Autodesk Fusion 360 part; units mm, degrees
(part 4 of 7)
  line L871 (67.0056, -68.9388) -> (67.1048, -68.852)
  line L872 (67.1048, -68.852) -> (67.2027, -68.7638)
  line L873 (67.2027, -68.7638) -> (67.2994, -68.6742)
  line L874 (67.2994, -68.6742) -> (67.2738, -68.5996)
  line L875 (67.2738, -68.5996) -> (67.2468, -68.526)
  line L876 (67.2468, -68.526) -> (67.2184, -68.4537)
  line L877 (67.2184, -68.4537) -> (67.1886, -68.3826)
  line L878 (67.1886, -68.3826) -> (67.1574, -68.3128)
  line L879 (67.1574, -68.3128) -> (67.1246, -68.2444)
  line L880 (67.1246, -68.2444) -> (67.0902, -68.1774)
  line L881 (67.0902, -68.1774) -> (67.0542, -68.1121)
  line L882 (67.0542, -68.1121) -> (67.0162, -68.0485)
  line L883 (67.0162, -68.0485) -> (66.9762, -67.987)
  line L884 (66.9762, -67.987) -> (66.9336, -67.9279)
  line L885 (66.9336, -67.9279) -> (66.8873, -67.8725)
  line L886 (66.8873, -67.8725) -> (66.5717, -67.5557)
  line L887 (66.5717, -67.5557) -> (66.7231, -67.4007)
  line L888 (66.7231, -67.4007) -> (66.8702, -67.2417)
  line L889 (66.8702, -67.2417) -> (67.013, -67.0787)
  line L890 (67.013, -67.0787) -> (67.1514, -66.9119)
  line L891 (67.1514, -66.9119) -> (67.4994, -67.1928)
  line L892 (67.4994, -67.1928) -> (67.5593, -67.233)
  line L893 (67.5593, -67.233) -> (67.6225, -67.2692)
  line L894 (67.6225, -67.2692) -> (67.6879, -67.3025)
  line L895 (67.6879, -67.3025) -> (67.7551, -67.3336)
  line L896 (67.7551, -67.3336) -> (67.8238, -67.3627)
  line L897 (67.8238, -67.3627) -> (67.894, -67.3899)
  line L898 (67.894, -67.3899) -> (67.9655, -67.4153)
  line L899 (67.9655, -67.4153) -> (68.0382, -67.4391)
  line L900 (68.0382, -67.4391) -> (68.112, -67.4613)
  line L901 (68.112, -67.4613) -> (68.1869, -67.4819)
  line L902 (68.1869, -67.4819) -> (68.2629, -67.5011)
  line L903 (68.2629, -67.5011) -> (68.3398, -67.5188)
  line L904 (68.3398, -67.5188) -> (68.4187, -67.4133)
  line L905 (68.4187, -67.4133) -> (68.4962, -67.3066)
  line L906 (68.4962, -67.3066) -> (68.5722, -67.1989)
  line L907 (68.5722, -67.1989) -> (68.5316, -67.1312)
  line L908 (68.5316, -67.1312) -> (68.4899, -67.0649)
  line L909 (68.4899, -67.0649) -> (68.4471, -67.0001)
  line L910 (68.4471, -67.0001) -> (68.4032, -66.9367)
  line L911 (68.4032, -66.9367) -> (68.3581, -66.8749)
  line L912 (68.3581, -66.8749) -> (68.3118, -66.8148)
  line L913 (68.3118, -66.8148) -> (68.2643, -66.7565)
  line L914 (68.2643, -66.7565) -> (68.2154, -66.7001)
  line L915 (68.2154, -66.7001) -> (68.1651, -66.6458)
  line L916 (68.1651, -66.6458) -> (68.1131, -66.5939)
  line L917 (68.1131, -66.5939) -> (68.0592, -66.545)
  line L918 (68.0592, -66.545) -> (68.0024, -66.5004)
  line L919 (68.0024, -66.5004) -> (67.6277, -66.2562)
  line L920 (67.6277, -66.2562) -> (67.7436, -66.0731)
  line L921 (67.7436, -66.0731) -> (67.8545, -65.8869)
  line L922 (67.8545, -65.8869) -> (67.9603, -65.6978)
  line L923 (67.9603, -65.6978) -> (68.0609, -65.5059)
  line L924 (68.0609, -65.5059) -> (68.4598, -65.7083)
  line L925 (68.4598, -65.7083) -> (68.5267, -65.7352)
  line L926 (68.5267, -65.7352) -> (68.5961, -65.7574)
  line L927 (68.5961, -65.7574) -> (68.667, -65.7765)
  line L928 (68.667, -65.7765) -> (68.7391, -65.7929)
  line L929 (68.7391, -65.7929) -> (68.8124, -65.807)
  line L930 (68.8124, -65.807) -> (68.8867, -65.819)
  line L931 (68.8867, -65.819) -> (68.9619, -65.8291)
  line L932 (68.9619, -65.8291) -> (69.038, -65.8372)
  line L933 (69.038, -65.8372) -> (69.1148, -65.8436)
  line L934 (69.1148, -65.8436) -> (69.1924, -65.8482)
  line L935 (69.1924, -65.8482) -> (69.2706, -65.8511)
  line L936 (69.2706, -65.8511) -> (69.3495, -65.8525)
  line L937 (69.3495, -65.8525) -> (69.4049, -65.7328)
  line L938 (69.4049, -65.7328) -> (69.4585, -65.6124)
  line L939 (69.4585, -65.6124) -> (69.5104, -65.4913)
  line L940 (69.5104, -65.4913) -> (69.4566, -65.4335)
  line L941 (69.4566, -65.4335) -> (69.402, -65.3773)
  line L942 (69.402, -65.3773) -> (69.3467, -65.3228)
  line L943 (69.3467, -65.3228) -> (69.2906, -65.2699)
  line L944 (69.2906, -65.2699) -> (69.2336, -65.2189)
  line L945 (69.2336, -65.2189) -> (69.1758, -65.1697)
  line L946 (69.1758, -65.1697) -> (69.1172, -65.1225)
  line L947 (69.1172, -65.1225) -> (69.0577, -65.0775)
  line L948 (69.0577, -65.0775) -> (68.9971, -65.0349)
  line L949 (68.9971, -65.0349) -> (68.9355, -64.9949)
  line L950 (68.9355, -64.9949) -> (68.8726, -64.9583)
  line L951 (68.8726, -64.9583) -> (68.8078, -64.9265)
  line L952 (68.8078, -64.9265) -> (68.3906, -64.7655)
  line L953 (68.3906, -64.7655) -> (68.4658, -64.5623)
  line L954 (68.4658, -64.5623) -> (68.5356, -64.3572)
  line L955 (68.5356, -64.3572) -> (68.5998, -64.1502)
  line L956 (68.5998, -64.1502) -> (68.6583, -63.9416)
  line L957 (68.6583, -63.9416) -> (69.0905, -64.0566)
  line L958 (69.0905, -64.0566) -> (69.1616, -64.069)
  line L959 (69.1616, -64.069) -> (69.234, -64.0763)
  line L960 (69.234, -64.0763) -> (69.3073, -64.0802)
  line L961 (69.3073, -64.0802) -> (69.3814, -64.0813)
  line L962 (69.3814, -64.0813) -> (69.456, -64.0798)
  line L963 (69.456, -64.0798) -> (69.5312, -64.0761)
  line L964 (69.5312, -64.0761) -> (69.6068, -64.0703)
  line L965 (69.6068, -64.0703) -> (69.6829, -64.0625)
  line L966 (69.6829, -64.0625) -> (69.7594, -64.0527)
  line L967 (69.7594, -64.0527) -> (69.8362, -64.0411)
  line L968 (69.8362, -64.0411) -> (69.9133, -64.0277)
  line L969 (69.9133, -64.0277) -> (69.9908, -64.0126)
  line L970 (69.9908, -64.0126) -> (70.02, -63.8841)
  line L971 (70.02, -63.8841) -> (70.0474, -63.7552)
  line L972 (70.0474, -63.7552) -> (70.073, -63.6259)
  line L973 (70.073, -63.6259) -> (70.0084, -63.5805)
  line L974 (70.0084, -63.5805) -> (69.9433, -63.5369)
  line L975 (69.9433, -63.5369) -> (69.8779, -63.4951)
  line L976 (69.8779, -63.4951) -> (69.812, -63.4551)
  line L977 (69.812, -63.4551) -> (69.7457, -63.417)
  line L978 (69.7457, -63.417) -> (69.6789, -63.3809)
  line L979 (69.6789, -63.3809) -> (69.6118, -63.3469)
  line L980 (69.6118, -63.3469) -> (69.5442, -63.3153)
  line L981 (69.5442, -63.3153) -> (69.4761, -63.2861)
  line L982 (69.4761, -63.2861) -> (69.4076, -63.2599)
  line L983 (69.4076, -63.2599) -> (69.3384, -63.2371)
  line L984 (69.3384, -63.2371) -> (69.2684, -63.2195)
  line L985 (69.2684, -63.2195) -> (68.8268, -63.1488)
  line L986 (68.8268, -63.1488) -> (68.8582, -62.9344)
  line L987 (68.8582, -62.9344) -> (68.8837, -62.7192)
  line L988 (68.8837, -62.7192) -> (68.9035, -62.5034)
  line L989 (68.9035, -62.5034) -> (68.9174, -62.2872)
  circle A0 centre (60.9176, -61.8819) radius 2
extrude "Extrude1''" add sketch "Sketch1 (3)" along normal blind 2 separate body makes body 5 in component "CT idler 2"
ref_plane "WorkPlane2" through (0, 0, 41.2) normal (0, 0, 1) x (1, 0, 0) in component "CT idler 2"
sketch "Sketch2 (2)" plane through (0, 0, 41.2) normal (0, 0, 1) x (1, 0, 0) in component "CT idler 2"
  line L0 (63.9717, -62.352) -> (64.2611, -62.3965)
  line L1 (64.2611, -62.3965) -> (64.3324, -62.3976)
  line L2 (64.3324, -62.3976) -> (64.4048, -62.3905)
  line L3 (64.4048, -62.3905) -> (64.478, -62.3776)
  line L4 (64.478, -62.3776) -> (64.5516, -62.3599)
  line L5 (64.5516, -62.3599) -> (64.6256, -62.3378)
  line L6 (64.6256, -62.3378) -> (64.6997, -62.3116)
  line L7 (64.6997, -62.3116) -> (64.774, -62.2814)
  line L8 (64.774, -62.2814) -> (64.8483, -62.2475)
  line L9 (64.8483, -62.2475) -> (64.9224, -62.21)
  line L10 (64.9224, -62.21) -> (64.9964, -62.1689)
  line L11 (64.9964, -62.1689) -> (65.07, -62.1243)
  line L12 (65.07, -62.1243) -> (65.1432, -62.0763)
  line L13 (65.1432, -62.0763) -> (65.1471, -61.9467)
  line L14 (65.1471, -61.9467) -> (65.1471, -61.8171)
  line L15 (65.1471, -61.8171) -> (65.1432, -61.6876)
  line L16 (65.1432, -61.6876) -> (65.07, -61.6396)
  line L17 (65.07, -61.6396) -> (64.9964, -61.595)
  line L18 (64.9964, -61.595) -> (64.9224, -61.5539)
  line L19 (64.9224, -61.5539) -> (64.8483, -61.5163)
  line L20 (64.8483, -61.5163) -> (64.774, -61.4824)
  line L21 (64.774, -61.4824) -> (64.6997, -61.4523)
  line L22 (64.6997, -61.4523) -> (64.6256, -61.4261)
  line L23 (64.6256, -61.4261) -> (64.5516, -61.404)
  line L24 (64.5516, -61.404) -> (64.478, -61.3862)
  line L25 (64.478, -61.3862) -> (64.4048, -61.3734)
  line L26 (64.4048, -61.3734) -> (64.3324, -61.3662)
  line L27 (64.3324, -61.3662) -> (64.2611, -61.3673)
  line L28 (64.2611, -61.3673) -> (63.9717, -61.4119)
  line L29 (63.9717, -61.4119) -> (63.9415, -61.2461)
  line L30 (63.9415, -61.2461) -> (63.9023, -61.0822)
  line L31 (63.9023, -61.0822) -> (63.8543, -60.9206)
  line L32 (63.8543, -60.9206) -> (63.7975, -60.762)
  line L33 (63.7975, -60.762) -> (64.0705, -60.6558)
  line L34 (64.0705, -60.6558) -> (64.1328, -60.6212)
  line L35 (64.1328, -60.6212) -> (64.1919, -60.5788)
  line L36 (64.1919, -60.5788) -> (64.2488, -60.5311)
  line L37 (64.2488, -60.5311) -> (64.3037, -60.4789)
  line L38 (64.3037, -60.4789) -> (64.3567, -60.4227)
  line L39 (64.3567, -60.4227) -> (64.4079, -60.3629)
  line L40 (64.4079, -60.3629) -> (64.4571, -60.2997)
  line L41 (64.4571, -60.2997) -> (64.5045, -60.2332)
  line L42 (64.5045, -60.2332) -> (64.5499, -60.1636)
  line L43 (64.5499, -60.1636) -> (64.5934, -60.0911)
  line L44 (64.5934, -60.0911) -> (64.6348, -60.0156)
  line L45 (64.6348, -60.0156) -> (64.6742, -59.9375)
  line L46 (64.6742, -59.9375) -> (64.6129, -59.8233)
  line L47 (64.6129, -59.8233) -> (64.5481, -59.7111)
  line L48 (64.5481, -59.7111) -> (64.4799, -59.6008)
  line L49 (64.4799, -59.6008) -> (64.3925, -59.5959)
  line L50 (64.3925, -59.5959) -> (64.3064, -59.5941)
  line L51 (64.3064, -59.5941) -> (64.2219, -59.5954)
  line L52 (64.2219, -59.5954) -> (64.1389, -59.6)
  line L53 (64.1389, -59.6) -> (64.0576, -59.6078)
  line L54 (64.0576, -59.6078) -> (63.9782, -59.6188)
  line L55 (63.9782, -59.6188) -> (63.9009, -59.6332)
  line L56 (63.9009, -59.6332) -> (63.8257, -59.651)
  line L57 (63.8257, -59.651) -> (63.7531, -59.6725)
  line L58 (63.7531, -59.6725) -> (63.6833, -59.6979)
  line L59 (63.6833, -59.6979) -> (63.617, -59.7279)
  line L60 (63.617, -59.7279) -> (63.5559, -59.7645)
  line L61 (63.5559, -59.7645) -> (63.3275, -59.9478)
  line L62 (63.3275, -59.9478) -> (63.2185, -59.8193)
  line L63 (63.2185, -59.8193) -> (63.1026, -59.697)
  line L64 (63.1026, -59.697) -> (62.9802, -59.5811)
  line L65 (62.9802, -59.5811) -> (62.8517, -59.4721)
  line L66 (62.8517, -59.4721) -> (63.035, -59.2436)
  line L67 (63.035, -59.2436) -> (63.0716, -59.1825)
  line L68 (63.0716, -59.1825) -> (63.1016, -59.1162)
  line L69 (63.1016, -59.1162) -> (63.1271, -59.0464)
  line L70 (63.1271, -59.0464) -> (63.1485, -58.9738)
  line L71 (63.1485, -58.9738) -> (63.1664, -58.8987)
  line L72 (63.1664, -58.8987) -> (63.1807, -58.8213)
  line L73 (63.1807, -58.8213) -> (63.1918, -58.7419)
  line L74 (63.1918, -58.7419) -> (63.1996, -58.6607)
  line L75 (63.1996, -58.6607) -> (63.2041, -58.5777)
  line L76 (63.2041, -58.5777) -> (63.2055, -58.4931)
  line L77 (63.2055, -58.4931) -> (63.2037, -58.4071)
  line L78 (63.2037, -58.4071) -> (63.1987, -58.3197)
  line L79 (63.1987, -58.3197) -> (63.0885, -58.2515)
  line L80 (63.0885, -58.2515) -> (62.9763, -58.1867)
  line L81 (62.9763, -58.1867) -> (62.8621, -58.1253)
  line L82 (62.8621, -58.1253) -> (62.7839, -58.1647)
  line L83 (62.7839, -58.1647) -> (62.7085, -58.2062)
  line L84 (62.7085, -58.2062) -> (62.6359, -58.2496)
  line L85 (62.6359, -58.2496) -> (62.5664, -58.2951)
  line L86 (62.5664, -58.2951) -> (62.4999, -58.3424)
  line L87 (62.4999, -58.3424) -> (62.4366, -58.3917)
  line L88 (62.4366, -58.3917) -> (62.3768, -58.4428)
  line L89 (62.3768, -58.4428) -> (62.3207, -58.4958)
  line L90 (62.3207, -58.4958) -> (62.2685, -58.5507)
  line L91 (62.2685, -58.5507) -> (62.2208, -58.6077)
  line L92 (62.2208, -58.6077) -> (62.1784, -58.6668)
  line L93 (62.1784, -58.6668) -> (62.1437, -58.7291)
  line L94 (62.1437, -58.7291) -> (62.0376, -59.002)
  line L95 (62.0376, -59.002) -> (61.8789, -58.9453)
  line L96 (61.8789, -58.9453) -> (61.7174, -58.8972)
  line L97 (61.7174, -58.8972) -> (61.5535, -58.8581)
  line L98 (61.5535, -58.8581) -> (61.3877, -58.8279)
  line L99 (61.3877, -58.8279) -> (61.4322, -58.5384)
  line L100 (61.4322, -58.5384) -> (61.4333, -58.4672)
  line L101 (61.4333, -58.4672) -> (61.4262, -58.3947)
  line L102 (61.4262, -58.3947) -> (61.4133, -58.3216)
  line L103 (61.4133, -58.3216) -> (61.3956, -58.248)
  line L104 (61.3956, -58.248) -> (61.3735, -58.174)
  line L105 (61.3735, -58.174) -> (61.3472, -58.0998)
  line L106 (61.3472, -58.0998) -> (61.3171, -58.0255)
  line L107 (61.3171, -58.0255) -> (61.2832, -57.9513)
  line L108 (61.2832, -57.9513) -> (61.2457, -57.8771)
  line L109 (61.2457, -57.8771) -> (61.2046, -57.8032)
  line L110 (61.2046, -57.8032) -> (61.16, -57.7296)
  line L111 (61.16, -57.7296) -> (61.112, -57.6564)
  line L112 (61.112, -57.6564) -> (60.9824, -57.6524)
  line L113 (60.9824, -57.6524) -> (60.8528, -57.6524)
  line L114 (60.8528, -57.6524) -> (60.7233, -57.6564)
  line L115 (60.7233, -57.6564) -> (60.6753, -57.7296)
  line L116 (60.6753, -57.7296) -> (60.6307, -57.8032)
  line L117 (60.6307, -57.8032) -> (60.5896, -57.8771)
  line L118 (60.5896, -57.8771) -> (60.552, -57.9513)
  line L119 (60.552, -57.9513) -> (60.5181, -58.0255)
  line L120 (60.5181, -58.0255) -> (60.488, -58.0998)
  line L121 (60.488, -58.0998) -> (60.4618, -58.174)
  line L122 (60.4618, -58.174) -> (60.4396, -58.248)
  line L123 (60.4396, -58.248) -> (60.4219, -58.3216)
  line L124 (60.4219, -58.3216) -> (60.4091, -58.3947)
  line L125 (60.4091, -58.3947) -> (60.4019, -58.4672)
  line L126 (60.4019, -58.4672) -> (60.403, -58.5384)
  line L127 (60.403, -58.5384) -> (60.4476, -58.8279)
  line L128 (60.4476, -58.8279) -> (60.2818, -58.8581)
  line L129 (60.2818, -58.8581) -> (60.1179, -58.8972)
  line L130 (60.1179, -58.8972) -> (59.9563, -58.9453)
  line L131 (59.9563, -58.9453) -> (59.7977, -59.002)
  line L132 (59.7977, -59.002) -> (59.6915, -58.7291)
  line L133 (59.6915, -58.7291) -> (59.6569, -58.6668)
  line L134 (59.6569, -58.6668) -> (59.6145, -58.6077)
  line L135 (59.6145, -58.6077) -> (59.5667, -58.5507)
  line L136 (59.5667, -58.5507) -> (59.5146, -58.4958)
  line L137 (59.5146, -58.4958) -> (59.4584, -58.4428)
  line L138 (59.4584, -58.4428) -> (59.3986, -58.3917)
  line L139 (59.3986, -58.3917) -> (59.3354, -58.3424)
  line L140 (59.3354, -58.3424) -> (59.2689, -58.2951)
  line L141 (59.2689, -58.2951) -> (59.1993, -58.2496)
  line L142 (59.1993, -58.2496) -> (59.1268, -58.2062)
  line L143 (59.1268, -58.2062) -> (59.0513, -58.1647)
  line L144 (59.0513, -58.1647) -> (58.9732, -58.1253)
  line L145 (58.9732, -58.1253) -> (58.859, -58.1867)
  line L146 (58.859, -58.1867) -> (58.7467, -58.2515)
  line L147 (58.7467, -58.2515) -> (58.6365, -58.3197)
  line L148 (58.6365, -58.3197) -> (58.6316, -58.4071)
  line L149 (58.6316, -58.4071) -> (58.6298, -58.4931)
  line L150 (58.6298, -58.4931) -> (58.6311, -58.5777)
  line L151 (58.6311, -58.5777) -> (58.6357, -58.6607)
  line L152 (58.6357, -58.6607) -> (58.6435, -58.7419)
  line L153 (58.6435, -58.7419) -> (58.6545, -58.8213)
  line L154 (58.6545, -58.8213) -> (58.6689, -58.8987)
  line L155 (58.6689, -58.8987) -> (58.6867, -58.9738)
  line L156 (58.6867, -58.9738) -> (58.7082, -59.0464)
  line L157 (58.7082, -59.0464) -> (58.7336, -59.1162)
  line L158 (58.7336, -59.1162) -> (58.7636, -59.1825)
  line L159 (58.7636, -59.1825) -> (58.8002, -59.2436)
  line L160 (58.8002, -59.2436) -> (58.9835, -59.4721)
  line L161 (58.9835, -59.4721) -> (58.855, -59.5811)
  line L162 (58.855, -59.5811) -> (58.7327, -59.697)
  line L163 (58.7327, -59.697) -> (58.6168, -59.8193)
  line L164 (58.6168, -59.8193) -> (58.5078, -59.9478)
  line L165 (58.5078, -59.9478) -> (58.2793, -59.7645)
  line L166 (58.2793, -59.7645) -> (58.2182, -59.7279)
  line L167 (58.2182, -59.7279) -> (58.1519, -59.6979)
  line L168 (58.1519, -59.6979) -> (58.0821, -59.6725)
  line L169 (58.0821, -59.6725) -> (58.0095, -59.651)
  line L170 (58.0095, -59.651) -> (57.9344, -59.6332)
  line L171 (57.9344, -59.6332) -> (57.857, -59.6188)
  line L172 (57.857, -59.6188) -> (57.7776, -59.6078)
  line L173 (57.7776, -59.6078) -> (57.6964, -59.6)
  line L174 (57.6964, -59.6) -> (57.6134, -59.5954)
  line L175 (57.6134, -59.5954) -> (57.5288, -59.5941)
  line L176 (57.5288, -59.5941) -> (57.4428, -59.5959)
  line L177 (57.4428, -59.5959) -> (57.3554, -59.6008)
  line L178 (57.3554, -59.6008) -> (57.2872, -59.7111)
  line L179 (57.2872, -59.7111) -> (57.2224, -59.8233)
  line L180 (57.2224, -59.8233) -> (57.161, -59.9375)
  line L181 (57.161, -59.9375) -> (57.2004, -60.0156)
  line L182 (57.2004, -60.0156) -> (57.2419, -60.0911)
  line L183 (57.2419, -60.0911) -> (57.2853, -60.1636)
  line L184 (57.2853, -60.1636) -> (57.3308, -60.2332)
  line L185 (57.3308, -60.2332) -> (57.3781, -60.2997)
  line L186 (57.3781, -60.2997) -> (57.4274, -60.3629)
  line L187 (57.4274, -60.3629) -> (57.4785, -60.4227)
  line L188 (57.4785, -60.4227) -> (57.5315, -60.4789)
  line L189 (57.5315, -60.4789) -> (57.5864, -60.5311)
  line L190 (57.5864, -60.5311) -> (57.6433, -60.5788)
  line L191 (57.6433, -60.5788) -> (57.7025, -60.6212)
  line L192 (57.7025, -60.6212) -> (57.7648, -60.6558)
  line L193 (57.7648, -60.6558) -> (58.0377, -60.762)
  line L194 (58.0377, -60.762) -> (57.981, -60.9206)
  line L195 (57.981, -60.9206) -> (57.9329, -61.0822)
  line L196 (57.9329, -61.0822) -> (57.8938, -61.2461)
  line L197 (57.8938, -61.2461) -> (57.8636, -61.4119)
  line L198 (57.8636, -61.4119) -> (57.5741, -61.3673)
  line L199 (57.5741, -61.3673) -> (57.5029, -61.3662)
  line L200 (57.5029, -61.3662) -> (57.4304, -61.3734)
  line L201 (57.4304, -61.3734) -> (57.3573, -61.3862)
  line L202 (57.3573, -61.3862) -> (57.2837, -61.404)
  line L203 (57.2837, -61.404) -> (57.2097, -61.4261)
  line L204 (57.2097, -61.4261) -> (57.1355, -61.4523)
  line L205 (57.1355, -61.4523) -> (57.0612, -61.4824)
  line L206 (57.0612, -61.4824) -> (56.987, -61.5163)
  line L207 (56.987, -61.5163) -> (56.9128, -61.5539)
  line L208 (56.9128, -61.5539) -> (56.8389, -61.595)
  line L209 (56.8389, -61.595) -> (56.7653, -61.6396)
  line L210 (56.7653, -61.6396) -> (56.6921, -61.6876)
  line L211 (56.6921, -61.6876) -> (56.6881, -61.8171)
  line L212 (56.6881, -61.8171) -> (56.6881, -61.9467)
  line L213 (56.6881, -61.9467) -> (56.6921, -62.0763)
  line L214 (56.6921, -62.0763) -> (56.7653, -62.1243)
  line L215 (56.7653, -62.1243) -> (56.8389, -62.1689)
  line L216 (56.8389, -62.1689) -> (56.9128, -62.21)
  line L217 (56.9128, -62.21) -> (56.987, -62.2475)
  line L218 (56.987, -62.2475) -> (57.0612, -62.2814)
  line L219 (57.0612, -62.2814) -> (57.1355, -62.3116)
  line L220 (57.1355, -62.3116) -> (57.2097, -62.3378)
  line L221 (57.2097, -62.3378) -> (57.2837, -62.3599)
  line L222 (57.2837, -62.3599) -> (57.3573, -62.3776)
  line L223 (57.3573, -62.3776) -> (57.4304, -62.3905)
  line L224 (57.4304, -62.3905) -> (57.5029, -62.3976)
  line L225 (57.5029, -62.3976) -> (57.5741, -62.3965)
  line L226 (57.5741, -62.3965) -> (57.8636, -62.352)
  line L227 (57.8636, -62.352) -> (57.8938, -62.5178)
  line L228 (57.8938, -62.5178) -> (57.9329, -62.6817)
  line L229 (57.9329, -62.6817) -> (57.981, -62.8432)
  line L230 (57.981, -62.8432) -> (58.0377, -63.0019)
  line L231 (58.0377, -63.0019) -> (57.7648, -63.108)
  line L232 (57.7648, -63.108) -> (57.7025, -63.1427)
  line L233 (57.7025, -63.1427) -> (57.6433, -63.1851)
  line L234 (57.6433, -63.1851) -> (57.5864, -63.2328)
  line L235 (57.5864, -63.2328) -> (57.5315, -63.285)
  line L236 (57.5315, -63.285) -> (57.4785, -63.3411)
  line L237 (57.4785, -63.3411) -> (57.4274, -63.4009)
  line L238 (57.4274, -63.4009) -> (57.3781, -63.4642)
  line L239 (57.3781, -63.4642) -> (57.3308, -63.5307)
  line L240 (57.3308, -63.5307) -> (57.2853, -63.6002)
  line L241 (57.2853, -63.6002) -> (57.2419, -63.6728)
  line L242 (57.2419, -63.6728) -> (57.2004, -63.7482)
  line L243 (57.2004, -63.7482) -> (57.161, -63.8264)
  line L244 (57.161, -63.8264) -> (57.2224, -63.9406)
  line L245 (57.2224, -63.9406) -> (57.2872, -64.0528)
  line L246 (57.2872, -64.0528) -> (57.3554, -64.163)
  line L247 (57.3554, -64.163) -> (57.4428, -64.168)
  line L248 (57.4428, -64.168) -> (57.5288, -64.1698)
  line L249 (57.5288, -64.1698) -> (57.6134, -64.1684)
  line L250 (57.6134, -64.1684) -> (57.6964, -64.1639)
  line L251 (57.6964, -64.1639) -> (57.7776, -64.1561)
  line L252 (57.7776, -64.1561) -> (57.857, -64.1451)
  line L253 (57.857, -64.1451) -> (57.9344, -64.1307)
  line L254 (57.9344, -64.1307) -> (58.0095, -64.1129)
  line L255 (58.0095, -64.1129) -> (58.0821, -64.0914)
  line L256 (58.0821, -64.0914) -> (58.1519, -64.066)
  line L257 (58.1519, -64.066) -> (58.2182, -64.0359)
  line L258 (58.2182, -64.0359) -> (58.2793, -63.9993)
  line L259 (58.2793, -63.9993) -> (58.5078, -63.816)
  line L260 (58.5078, -63.816) -> (58.6168, -63.9445)
  line L261 (58.6168, -63.9445) -> (58.7327, -64.0669)
  line L262 (58.7327, -64.0669) -> (58.855, -64.1828)
  line L263 (58.855, -64.1828) -> (58.9835, -64.2918)
  line L264 (58.9835, -64.2918) -> (58.8002, -64.5202)
  line L265 (58.8002, -64.5202) -> (58.7636, -64.5813)
  line L266 (58.7636, -64.5813) -> (58.7336, -64.6476)
  line L267 (58.7336, -64.6476) -> (58.7082, -64.7174)
  line L268 (58.7082, -64.7174) -> (58.6867, -64.79)
  line L269 (58.6867, -64.79) -> (58.6689, -64.8652)
  line L270 (58.6689, -64.8652) -> (58.6545, -64.9425)
  line L271 (58.6545, -64.9425) -> (58.6435, -65.0219)
  line L272 (58.6435, -65.0219) -> (58.6357, -65.1032)
  line L273 (58.6357, -65.1032) -> (58.6311, -65.1862)
  line L274 (58.6311, -65.1862) -> (58.6298, -65.2707)
  line L275 (58.6298, -65.2707) -> (58.6316, -65.3568)
  line L276 (58.6316, -65.3568) -> (58.6365, -65.4442)
  line L277 (58.6365, -65.4442) -> (58.7467, -65.5124)
  line L278 (58.7467, -65.5124) -> (58.859, -65.5772)
  line L279 (58.859, -65.5772) -> (58.9732, -65.6385)
  line L280 (58.9732, -65.6385) -> (59.0513, -65.5991)
  line L281 (59.0513, -65.5991) -> (59.1268, -65.5577)
  line L282 (59.1268, -65.5577) -> (59.1993, -65.5142)
  line L283 (59.1993, -65.5142) -> (59.2689, -65.4688)
  line L284 (59.2689, -65.4688) -> (59.3354, -65.4214)
  line L285 (59.3354, -65.4214) -> (59.3986, -65.3722)
  line L286 (59.3986, -65.3722) -> (59.4584, -65.321)
  line L287 (59.4584, -65.321) -> (59.5146, -65.268)
  line L288 (59.5146, -65.268) -> (59.5667, -65.2131)
  line L289 (59.5667, -65.2131) -> (59.6145, -65.1562)
  line L290 (59.6145, -65.1562) -> (59.6569, -65.0971)
  line L291 (59.6569, -65.0971) -> (59.6915, -65.0348)
  line L292 (59.6915, -65.0348) -> (59.7977, -64.7618)
  line L293 (59.7977, -64.7618) -> (59.9563, -64.8186)
  line L294 (59.9563, -64.8186) -> (60.1179, -64.8666)
  line L295 (60.1179, -64.8666) -> (60.2818, -64.9058)
  line L296 (60.2818, -64.9058) -> (60.4476, -64.936)
  line L297 (60.4476, -64.936) -> (60.403, -65.2255)
  line L298 (60.403, -65.2255) -> (60.4019, -65.2967)
  line L299 (60.4019, -65.2967) -> (60.4091, -65.3691)
  line L300 (60.4091, -65.3691) -> (60.4219, -65.4423)
  line L301 (60.4219, -65.4423) -> (60.4396, -65.5159)
  line L302 (60.4396, -65.5159) -> (60.4618, -65.5899)
  line L303 (60.4618, -65.5899) -> (60.488, -65.6641)
  line L304 (60.488, -65.6641) -> (60.5181, -65.7383)
  line L305 (60.5181, -65.7383) -> (60.552, -65.8126)
  line L306 (60.552, -65.8126) -> (60.5896, -65.8867)
  line L307 (60.5896, -65.8867) -> (60.6307, -65.9607)
  line L308 (60.6307, -65.9607) -> (60.6753, -66.0343)
  line L309 (60.6753, -66.0343) -> (60.7233, -66.1075)
  line L310 (60.7233, -66.1075) -> (60.8528, -66.1114)
  line L311 (60.8528, -66.1114) -> (60.9824, -66.1114)
  line L312 (60.9824, -66.1114) -> (61.112, -66.1075)
  line L313 (61.112, -66.1075) -> (61.16, -66.0343)
  line L314 (61.16, -66.0343) -> (61.2046, -65.9607)
  line L315 (61.2046, -65.9607) -> (61.2457, -65.8867)
  line L316 (61.2457, -65.8867) -> (61.2832, -65.8126)
  line L317 (61.2832, -65.8126) -> (61.3171, -65.7383)
  line L318 (61.3171, -65.7383) -> (61.3472, -65.6641)
  line L319 (61.3472, -65.6641) -> (61.3735, -65.5899)
  line L320 (61.3735, -65.5899) -> (61.3956, -65.5159)
  line L321 (61.3956, -65.5159) -> (61.4133, -65.4423)
  line L322 (61.4133, -65.4423) -> (61.4262, -65.3691)
  line L323 (61.4262, -65.3691) -> (61.4333, -65.2967)
  line L324 (61.4333, -65.2967) -> (61.4322, -65.2255)
  line L325 (61.4322, -65.2255) -> (61.3877, -64.936)
  line L326 (61.3877, -64.936) -> (61.5535, -64.9058)
  line L327 (61.5535, -64.9058) -> (61.7174, -64.8666)
  line L328 (61.7174, -64.8666) -> (61.8789, -64.8186)
  line L329 (61.8789, -64.8186) -> (62.0376, -64.7618)
  line L330 (62.0376, -64.7618) -> (62.1437, -65.0348)
  line L331 (62.1437, -65.0348) -> (62.1784, -65.0971)
  line L332 (62.1784, -65.0971) -> (62.2208, -65.1562)
  line L333 (62.2208, -65.1562) -> (62.2685, -65.2131)
  line L334 (62.2685, -65.2131) -> (62.3207, -65.268)
  line L335 (62.3207, -65.268) -> (62.3768, -65.321)
  line L336 (62.3768, -65.321) -> (62.4366, -65.3722)
  line L337 (62.4366, -65.3722) -> (62.4999, -65.4214)
  line L338 (62.4999, -65.4214) -> (62.5664, -65.4688)
  line L339 (62.5664, -65.4688) -> (62.6359, -65.5142)
  line L340 (62.6359, -65.5142) -> (62.7085, -65.5577)
  line L341 (62.7085, -65.5577) -> (62.7839, -65.5991)
  line L342 (62.7839, -65.5991) -> (62.8621, -65.6385)
  line L343 (62.8621, -65.6385) -> (62.9763, -65.5772)
  line L344 (62.9763, -65.5772) -> (63.0885, -65.5124)
  line L345 (63.0885, -65.5124) -> (63.1987, -65.4442)
  line L346 (63.1987, -65.4442) -> (63.2037, -65.3568)
  line L347 (63.2037, -65.3568) -> (63.2055, -65.2707)
  line L348 (63.2055, -65.2707) -> (63.2041, -65.1862)
  line L349 (63.2041, -65.1862) -> (63.1996, -65.1032)
  line L350 (63.1996, -65.1032) -> (63.1918, -65.0219)
  line L351 (63.1918, -65.0219) -> (63.1807, -64.9425)
  line L352 (63.1807, -64.9425) -> (63.1664, -64.8652)
  line L353 (63.1664, -64.8652) -> (63.1485, -64.79)
  line L354 (63.1485, -64.79) -> (63.1271, -64.7174)
  line L355 (63.1271, -64.7174) -> (63.1016, -64.6476)
  line L356 (63.1016, -64.6476) -> (63.0716, -64.5813)
  line L357 (63.0716, -64.5813) -> (63.035, -64.5202)
  line L358 (63.035, -64.5202) -> (62.8517, -64.2918)
  line L359 (62.8517, -64.2918) -> (62.9802, -64.1828)
  line L360 (62.9802, -64.1828) -> (63.1026, -64.0669)
  line L361 (63.1026, -64.0669) -> (63.2185, -63.9445)
  line L362 (63.2185, -63.9445) -> (63.3275, -63.816)
  line L363 (63.3275, -63.816) -> (63.5559, -63.9993)
  line L364 (63.5559, -63.9993) -> (63.617, -64.0359)
  line L365 (63.617, -64.0359) -> (63.6833, -64.066)
  line L366 (63.6833, -64.066) -> (63.7531, -64.0914)
  line L367 (63.7531, -64.0914) -> (63.8257, -64.1129)
  line L368 (63.8257, -64.1129) -> (63.9009, -64.1307)
  line L369 (63.9009, -64.1307) -> (63.9782, -64.1451)
  line L370 (63.9782, -64.1451) -> (64.0576, -64.1561)
  line L371 (64.0576, -64.1561) -> (64.1389, -64.1639)
  line L372 (64.1389, -64.1639) -> (64.2219, -64.1684)
  line L373 (64.2219, -64.1684) -> (64.3064, -64.1698)
  line L374 (64.3064, -64.1698) -> (64.3925, -64.168)
  line L375 (64.3925, -64.168) -> (64.4799, -64.163)
  line L376 (64.4799, -64.163) -> (64.5481, -64.0528)
  line L377 (64.5481, -64.0528) -> (64.6129, -63.9406)
  line L378 (64.6129, -63.9406) -> (64.6742, -63.8264)
  line L379 (64.6742, -63.8264) -> (64.6348, -63.7482)
  line L380 (64.6348, -63.7482) -> (64.5934, -63.6728)
  line L381 (64.5934, -63.6728) -> (64.5499, -63.6002)
  line L382 (64.5499, -63.6002) -> (64.5045, -63.5307)
  line L383 (64.5045, -63.5307) -> (64.4571, -63.4642)
  line L384 (64.4571, -63.4642) -> (64.4079, -63.4009)
  line L385 (64.4079, -63.4009) -> (64.3567, -63.3411)
  line L386 (64.3567, -63.3411) -> (64.3037, -63.285)
  line L387 (64.3037, -63.285) -> (64.2488, -63.2328)
  line L388 (64.2488, -63.2328) -> (64.1919, -63.1851)
  line L389 (64.1919, -63.1851) -> (64.1328, -63.1427)
  line L390 (64.1328, -63.1427) -> (64.0705, -63.108)
  line L391 (64.0705, -63.108) -> (63.7975, -63.0019)
  line L392 (63.7975, -63.0019) -> (63.8543, -62.8432)
  line L393 (63.8543, -62.8432) -> (63.9023, -62.6817)
  line L394 (63.9023, -62.6817) -> (63.9415, -62.5178)
  line L395 (63.9415, -62.5178) -> (63.9717, -62.352)
  circle A0 centre (60.9176, -61.8819) radius 2
extrude "Extrude2'" add sketch "Sketch2 (2)" along normal blind 2 separate body makes body 6 in component "CT idler 2"
combine "Combine1'" operation add target body 5 tool bodies 6 makes body 7 at (62.269, -64.2225, 41.2) in component "CT idler 2"
ref_plane "WorkPlane1" through (0, 0, 41.2) normal (0, 0, 1) x (1, 0, 0) in component "CT idler 3"
sketch "Sketch1 (4)" plane through (0, 0, 41.2) normal (0, 0, 1) x (1, 0, 0) in component "CT idler 3"
  line L0 (72.6863, -50.2641) -> (73.133, -50.2867)
  line L1 (73.133, -50.2867) -> (73.2051, -50.2841)
  line L2 (73.2051, -50.2841) -> (73.2775, -50.2762)
  line L3 (73.2775, -50.2762) -> (73.35, -50.2647)
  line L4 (73.35, -50.2647) -> (73.4226, -50.2504)
  line L5 (73.4226, -50.2504) -> (73.4953, -50.2335)
  line L6 (73.4953, -50.2335) -> (73.5681, -50.2142)
  line L7 (73.5681, -50.2142) -> (73.6409, -50.1928)
  line L8 (73.6409, -50.1928) -> (73.7137, -50.1693)
  line L9 (73.7137, -50.1693) -> (73.7864, -50.1439)
  line L10 (73.7864, -50.1439) -> (73.8592, -50.1166)
  line L11 (73.8592, -50.1166) -> (73.9319, -50.0874)
  line L12 (73.9319, -50.0874) -> (74.0045, -50.0565)
  line L13 (74.0045, -50.0565) -> (74.0064, -49.9247)
  line L14 (74.0064, -49.9247) -> (74.0064, -49.7929)
  line L15 (74.0064, -49.7929) -> (74.0045, -49.6611)
  line L16 (74.0045, -49.6611) -> (73.9319, -49.6302)
  line L17 (73.9319, -49.6302) -> (73.8592, -49.6011)
  line L18 (73.8592, -49.6011) -> (73.7864, -49.5738)
  line L19 (73.7864, -49.5738) -> (73.7137, -49.5483)
  line L20 (73.7137, -49.5483) -> (73.6409, -49.5249)
  line L21 (73.6409, -49.5249) -> (73.5681, -49.5034)
  line L22 (73.5681, -49.5034) -> (73.4953, -49.4842)
  line L23 (73.4953, -49.4842) -> (73.4226, -49.4673)
  line L24 (73.4226, -49.4673) -> (73.35, -49.4529)
  line L25 (73.35, -49.4529) -> (73.2775, -49.4415)
  line L26 (73.2775, -49.4415) -> (73.2051, -49.4336)
  line L27 (73.2051, -49.4336) -> (73.133, -49.431)
  line L28 (73.133, -49.431) -> (72.6863, -49.4536)
  line L29 (72.6863, -49.4536) -> (72.6724, -49.2373)
  line L30 (72.6724, -49.2373) -> (72.6527, -49.0216)
  line L31 (72.6527, -49.0216) -> (72.6271, -48.8064)
  line L32 (72.6271, -48.8064) -> (72.5958, -48.592)
  line L33 (72.5958, -48.592) -> (73.0374, -48.5212)
  line L34 (73.0374, -48.5212) -> (73.1074, -48.5037)
  line L35 (73.1074, -48.5037) -> (73.1765, -48.4809)
  line L36 (73.1765, -48.4809) -> (73.2451, -48.4546)
  line L37 (73.2451, -48.4546) -> (73.3131, -48.4255)
  line L38 (73.3131, -48.4255) -> (73.3807, -48.3938)
  line L39 (73.3807, -48.3938) -> (73.4479, -48.3599)
  line L40 (73.4479, -48.3599) -> (73.5146, -48.3238)
  line L41 (73.5146, -48.3238) -> (73.5809, -48.2857)
  line L42 (73.5809, -48.2857) -> (73.6468, -48.2457)
  line L43 (73.6468, -48.2457) -> (73.7123, -48.2038)
  line L44 (73.7123, -48.2038) -> (73.7774, -48.1602)
  line L45 (73.7774, -48.1602) -> (73.842, -48.1149)
  line L46 (73.842, -48.1149) -> (73.8164, -47.9856)
  line L47 (73.8164, -47.9856) -> (73.789, -47.8567)
  line L48 (73.789, -47.8567) -> (73.7598, -47.7282)
  line L49 (73.7598, -47.7282) -> (73.6823, -47.713)
  line L50 (73.6823, -47.713) -> (73.6051, -47.6997)
  line L51 (73.6051, -47.6997) -> (73.5283, -47.6881)
  line L52 (73.5283, -47.6881) -> (73.4518, -47.6783)
  line L53 (73.4518, -47.6783) -> (73.3758, -47.6705)
  line L54 (73.3758, -47.6705) -> (73.3001, -47.6646)
  line L55 (73.3001, -47.6646) -> (73.225, -47.6609)
  line L56 (73.225, -47.6609) -> (73.1503, -47.6595)
  line L57 (73.1503, -47.6595) -> (73.0763, -47.6606)
  line L58 (73.0763, -47.6606) -> (73.003, -47.6645)
  line L59 (73.003, -47.6645) -> (72.9305, -47.6718)
  line L60 (72.9305, -47.6718) -> (72.8595, -47.6842)
  line L61 (72.8595, -47.6842) -> (72.4273, -47.7992)
  line L62 (72.4273, -47.7992) -> (72.3687, -47.5906)
  line L63 (72.3687, -47.5906) -> (72.3045, -47.3836)
  line L64 (72.3045, -47.3836) -> (72.2348, -47.1784)
  line L65 (72.2348, -47.1784) -> (72.1595, -46.9753)
  line L66 (72.1595, -46.9753) -> (72.5768, -46.8142)
  line L67 (72.5768, -46.8142) -> (72.6416, -46.7825)
  line L68 (72.6416, -46.7825) -> (72.7045, -46.7458)
  line L69 (72.7045, -46.7458) -> (72.7661, -46.7059)
  line L70 (72.7661, -46.7059) -> (72.8266, -46.6633)
  line L71 (72.8266, -46.6633) -> (72.8862, -46.6182)
  line L72 (72.8862, -46.6182) -> (72.9448, -46.5711)
  line L73 (72.9448, -46.5711) -> (73.0026, -46.5219)
  line L74 (73.0026, -46.5219) -> (73.0595, -46.4708)
  line L75 (73.0595, -46.4708) -> (73.1156, -46.418)
  line L76 (73.1156, -46.418) -> (73.171, -46.3634)
  line L77 (73.171, -46.3634) -> (73.2255, -46.3073)
  line L78 (73.2255, -46.3073) -> (73.2793, -46.2495)
  line L79 (73.2793, -46.2495) -> (73.2274, -46.1283)
  line L80 (73.2274, -46.1283) -> (73.1738, -46.0079)
  line L81 (73.1738, -46.0079) -> (73.1185, -45.8883)
  line L82 (73.1185, -45.8883) -> (73.0396, -45.8896)
  line L83 (73.0396, -45.8896) -> (72.9613, -45.8926)
  line L84 (72.9613, -45.8926) -> (72.8838, -45.8972)
  line L85 (72.8838, -45.8972) -> (72.8069, -45.9035)
  line L86 (72.8069, -45.9035) -> (72.7309, -45.9117)
  line L87 (72.7309, -45.9117) -> (72.6557, -45.9217)
  line L88 (72.6557, -45.9217) -> (72.5814, -45.9337)
  line L89 (72.5814, -45.9337) -> (72.5081, -45.9479)
  line L90 (72.5081, -45.9479) -> (72.4359, -45.9643)
  line L91 (72.4359, -45.9643) -> (72.365, -45.9834)
  line L92 (72.365, -45.9834) -> (72.2957, -46.0056)
  line L93 (72.2957, -46.0056) -> (72.2287, -46.0325)
  line L94 (72.2287, -46.0325) -> (71.8299, -46.2348)
  line L95 (71.8299, -46.2348) -> (71.7292, -46.0429)
  line L96 (71.7292, -46.0429) -> (71.6234, -45.8538)
  line L97 (71.6234, -45.8538) -> (71.5126, -45.6677)
  line L98 (71.5126, -45.6677) -> (71.3967, -45.4845)
  line L99 (71.3967, -45.4845) -> (71.7714, -45.2403)
  line L100 (71.7714, -45.2403) -> (71.8282, -45.1958)
  line L101 (71.8282, -45.1958) -> (71.8821, -45.1469)
  line L102 (71.8821, -45.1469) -> (71.934, -45.095)
  line L103 (71.934, -45.095) -> (71.9843, -45.0407)
  line L104 (71.9843, -45.0407) -> (72.0332, -44.9843)
  line L105 (72.0332, -44.9843) -> (72.0808, -44.9259)
  line L106 (72.0808, -44.9259) -> (72.1271, -44.8658)
  line L107 (72.1271, -44.8658) -> (72.1721, -44.804)
  line L108 (72.1721, -44.804) -> (72.2161, -44.7407)
  line L109 (72.2161, -44.7407) -> (72.2588, -44.6758)
  line L110 (72.2588, -44.6758) -> (72.3005, -44.6095)
  line L111 (72.3005, -44.6095) -> (72.3411, -44.5418)
  line L112 (72.3411, -44.5418) -> (72.2652, -44.4341)
  line L113 (72.2652, -44.4341) -> (72.1877, -44.3275)
  line L114 (72.1877, -44.3275) -> (72.1087, -44.222)
  line L115 (72.1087, -44.222) -> (72.0318, -44.2397)
  line L116 (72.0318, -44.2397) -> (71.9559, -44.2588)
  line L117 (71.9559, -44.2588) -> (71.881, -44.2795)
  line L118 (71.881, -44.2795) -> (71.8071, -44.3017)
  line L119 (71.8071, -44.3017) -> (71.7345, -44.3254)
  line L120 (71.7345, -44.3254) -> (71.663, -44.3509)
  line L121 (71.663, -44.3509) -> (71.5928, -44.3781)
  line L122 (71.5928, -44.3781) -> (71.5241, -44.4071)
  line L123 (71.5241, -44.4071) -> (71.4569, -44.4382)
  line L124 (71.4569, -44.4382) -> (71.3915, -44.4716)
  line L125 (71.3915, -44.4716) -> (71.3283, -44.5077)
  line L126 (71.3283, -44.5077) -> (71.2684, -44.548)
  line L127 (71.2684, -44.548) -> (70.9203, -44.8289)
  line L128 (70.9203, -44.8289) -> (70.782, -44.6621)
  line L129 (70.782, -44.6621) -> (70.6392, -44.4991)
  line L130 (70.6392, -44.4991) -> (70.492, -44.34)
  line L131 (70.492, -44.34) -> (70.3406, -44.185)
  line L132 (70.3406, -44.185) -> (70.6563, -43.8682)
  line L133 (70.6563, -43.8682) -> (70.7026, -43.8129)
  line L134 (70.7026, -43.8129) -> (70.7452, -43.7538)
  line L135 (70.7452, -43.7538) -> (70.7852, -43.6922)
  line L136 (70.7852, -43.6922) -> (70.8231, -43.6287)
  line L137 (70.8231, -43.6287) -> (70.8592, -43.5633)
  line L138 (70.8592, -43.5633) -> (70.8936, -43.4964)
  line L139 (70.8936, -43.4964) -> (70.9264, -43.428)
  line L140 (70.9264, -43.428) -> (70.9576, -43.3582)
  line L141 (70.9576, -43.3582) -> (70.9874, -43.2871)
  line L142 (70.9874, -43.2871) -> (71.0158, -43.2147)
  line L143 (71.0158, -43.2147) -> (71.0428, -43.1412)
  line L144 (71.0428, -43.1412) -> (71.0684, -43.0666)
  line L145 (71.0684, -43.0666) -> (70.9717, -42.977)
  line L146 (70.9717, -42.977) -> (70.8738, -42.8888)
  line L147 (70.8738, -42.8888) -> (70.7746, -42.802)
  line L148 (70.7746, -42.802) -> (70.703, -42.8353)
  line L149 (70.703, -42.8353) -> (70.6327, -42.8698)
  line L150 (70.6327, -42.8698) -> (70.5637, -42.9056)
  line L151 (70.5637, -42.9056) -> (70.4961, -42.9427)
  line L152 (70.4961, -42.9427) -> (70.43, -42.981)
  line L153 (70.43, -42.981) -> (70.3654, -43.0208)
  line L154 (70.3654, -43.0208) -> (70.3024, -43.062)
  line L155 (70.3024, -43.062) -> (70.2412, -43.1047)
  line L156 (70.2412, -43.1047) -> (70.1819, -43.1491)
  line L157 (70.1819, -43.1491) -> (70.1249, -43.1953)
  line L158 (70.1249, -43.1953) -> (70.0706, -43.2438)
  line L159 (70.0706, -43.2438) -> (70.0204, -43.2956)
  line L160 (70.0204, -43.2956) -> (69.7383, -43.6427)
  line L161 (69.7383, -43.6427) -> (69.5683, -43.5083)
  line L162 (69.5683, -43.5083) -> (69.3947, -43.3786)
  line L163 (69.3947, -43.3786) -> (69.2177, -43.2536)
  line L164 (69.2177, -43.2536) -> (69.0374, -43.1335)
  line L165 (69.0374, -43.1335) -> (69.2803, -42.758)
  line L166 (69.2803, -42.758) -> (69.3141, -42.6942)
  line L167 (69.3141, -42.6942) -> (69.3435, -42.6276)
  line L168 (69.3435, -42.6276) -> (69.3698, -42.559)
  line L169 (69.3698, -42.559) -> (69.3937, -42.489)
  line L170 (69.3937, -42.489) -> (69.4154, -42.4175)
  line L171 (69.4154, -42.4175) -> (69.4351, -42.3449)
  line L172 (69.4351, -42.3449) -> (69.453, -42.2712)
  line L173 (69.453, -42.2712) -> (69.469, -42.1964)
  line L174 (69.469, -42.1964) -> (69.4834, -42.1207)
  line L175 (69.4834, -42.1207) -> (69.4961, -42.044)
  line L176 (69.4961, -42.044) -> (69.5072, -41.9665)
  line L177 (69.5072, -41.9665) -> (69.5167, -41.8881)
  line L178 (69.5167, -41.8881) -> (69.4035, -41.8206)
  line L179 (69.4035, -41.8206) -> (69.2894, -41.7547)
  line L180 (69.2894, -41.7547) -> (69.1743, -41.6904)
  line L181 (69.1743, -41.6904) -> (69.1113, -41.7379)
  line L182 (69.1113, -41.7379) -> (69.0497, -41.7863)
  line L183 (69.0497, -41.7863) -> (68.9897, -41.8356)
  line L184 (68.9897, -41.8356) -> (68.9312, -41.8859)
  line L185 (68.9312, -41.8859) -> (68.8745, -41.9372)
  line L186 (68.8745, -41.9372) -> (68.8196, -41.9895)
  line L187 (68.8196, -41.9895) -> (68.7665, -42.0429)
  line L188 (68.7665, -42.0429) -> (68.7155, -42.0974)
  line L189 (68.7155, -42.0974) -> (68.6668, -42.1531)
  line L190 (68.6668, -42.1531) -> (68.6206, -42.2102)
  line L191 (68.6206, -42.2102) -> (68.5776, -42.269)
  line L192 (68.5776, -42.269) -> (68.5392, -42.3301)
  line L193 (68.5392, -42.3301) -> (68.3355, -42.7282)
  line L194 (68.3355, -42.7282) -> (68.1413, -42.6321)
  line L195 (68.1413, -42.6321) -> (67.9445, -42.5413)
  line L196 (67.9445, -42.5413) -> (67.7454, -42.4559)
  line L197 (67.7454, -42.4559) -> (67.5441, -42.3759)
  line L198 (67.5441, -42.3759) -> (67.7036, -41.958)
  line L199 (67.7036, -41.958) -> (67.7234, -41.8886)
  line L200 (67.7234, -41.8886) -> (67.7382, -41.8174)
  line L201 (67.7382, -41.8174) -> (67.7498, -41.7449)
  line L202 (67.7498, -41.7449) -> (67.7586, -41.6713)
  line L203 (67.7586, -41.6713) -> (67.7649, -41.597)
  line L204 (67.7649, -41.597) -> (67.7691, -41.5218)
  line L205 (67.7691, -41.5218) -> (67.7712, -41.446)
  line L206 (67.7712, -41.446) -> (67.7714, -41.3695)
  line L207 (67.7714, -41.3695) -> (67.7697, -41.2924)
  line L208 (67.7697, -41.2924) -> (67.7662, -41.2148)
  line L209 (67.7662, -41.2148) -> (67.7609, -41.1367)
  line L210 (67.7609, -41.1367) -> (67.754, -41.0581)
  line L211 (67.754, -41.0581) -> (67.6292, -41.0156)
  line L212 (67.6292, -41.0156) -> (67.5039, -40.9748)
  line L213 (67.5039, -40.9748) -> (67.378, -40.9359)
  line L214 (67.378, -40.9359) -> (67.3261, -40.9954)
  line L215 (67.3261, -40.9954) -> (67.276, -41.0555)
  line L216 (67.276, -41.0555) -> (67.2275, -41.1163)
  line L217 (67.2275, -41.1163) -> (67.1808, -41.1776)
  line L218 (67.1808, -41.1776) -> (67.136, -41.2396)
  line L219 (67.136, -41.2396) -> (67.0931, -41.3022)
  line L220 (67.0931, -41.3022) -> (67.0523, -41.3654)
  line L221 (67.0523, -41.3654) -> (67.0138, -41.4294)
  line L222 (67.0138, -41.4294) -> (66.9777, -41.494)
  line L223 (66.9777, -41.494) -> (66.9444, -41.5594)
  line L224 (66.9444, -41.5594) -> (66.9145, -41.6258)
  line L225 (66.9145, -41.6258) -> (66.8897, -41.6936)
  line L226 (66.8897, -41.6936) -> (66.7732, -42.1254)
  line L227 (66.7732, -42.1254) -> (66.5633, -42.0718)
  line L228 (66.5633, -42.0718) -> (66.352, -42.0239)
  line L229 (66.352, -42.0239) -> (66.1394, -41.9817)
  line L230 (66.1394, -41.9817) -> (65.9258, -41.9453)
  line L231 (65.9258, -41.9453) -> (65.995, -41.5034)
  line L232 (65.995, -41.5034) -> (65.9999, -41.4314)
  line L233 (65.9999, -41.4314) -> (65.9996, -41.3586)
  line L234 (65.9996, -41.3586) -> (65.9958, -41.2853)
  line L235 (65.9958, -41.2853) -> (65.9892, -41.2116)
  line L236 (65.9892, -41.2116) -> (65.9799, -41.1375)
  line L237 (65.9799, -41.1375) -> (65.9684, -41.0631)
  line L238 (65.9684, -41.0631) -> (65.9547, -40.9885)
  line L239 (65.9547, -40.9885) -> (65.939, -40.9137)
  line L240 (65.939, -40.9137) -> (65.9213, -40.8386)
  line L241 (65.9213, -40.8386) -> (65.9017, -40.7634)
  line L242 (65.9017, -40.7634) -> (65.8803, -40.6881)
  line L243 (65.8803, -40.6881) -> (65.8572, -40.6126)
  line L244 (65.8572, -40.6126) -> (65.7263, -40.597)
  line L245 (65.7263, -40.597) -> (65.5952, -40.5832)
  line L246 (65.5952, -40.5832) -> (65.464, -40.5713)
  line L247 (65.464, -40.5713) -> (65.4256, -40.6403)
  line L248 (65.4256, -40.6403) -> (65.3891, -40.7096)
  line L249 (65.3891, -40.7096) -> (65.3543, -40.779)
  line L250 (65.3543, -40.779) -> (65.3214, -40.8488)
  line L251 (65.3214, -40.8488) -> (65.2904, -40.9187)
  line L252 (65.2904, -40.9187) -> (65.2615, -40.9888)
  line L253 (65.2615, -40.9888) -> (65.2348, -41.0592)
  line L254 (65.2348, -41.0592) -> (65.2103, -41.1297)
  line L255 (65.2103, -41.1297) -> (65.1885, -41.2004)
  line L256 (65.1885, -41.2004) -> (65.1695, -41.2714)
  line L257 (65.1695, -41.2714) -> (65.1541, -41.3425)
  line L258 (65.1541, -41.3425) -> (65.1439, -41.414)
  line L259 (65.1439, -41.414) -> (65.1198, -41.8606)
  line L260 (65.1198, -41.8606) -> (64.9033, -41.8518)
  line L261 (64.9033, -41.8518) -> (64.6866, -41.8488)
  line L262 (64.6866, -41.8488) -> (64.4699, -41.8518)
  line L263 (64.4699, -41.8518) -> (64.2534, -41.8606)
  line L264 (64.2534, -41.8606) -> (64.2292, -41.414)
  line L265 (64.2292, -41.414) -> (64.2191, -41.3425)
  line L266 (64.2191, -41.3425) -> (64.2036, -41.2714)
  line L267 (64.2036, -41.2714) -> (64.1847, -41.2004)
  line L268 (64.1847, -41.2004) -> (64.1628, -41.1297)
  line L269 (64.1628, -41.1297) -> (64.1384, -41.0592)
  line L270 (64.1384, -41.0592) -> (64.1117, -40.9888)
  line L271 (64.1117, -40.9888) -> (64.0827, -40.9187)
  line L272 (64.0827, -40.9187) -> (64.0518, -40.8488)
  line L273 (64.0518, -40.8488) -> (64.0189, -40.779)
  line L274 (64.0189, -40.779) -> (63.9841, -40.7096)
  line L275 (63.9841, -40.7096) -> (63.9475, -40.6403)
  line L276 (63.9475, -40.6403) -> (63.9092, -40.5713)
  line L277 (63.9092, -40.5713) -> (63.7779, -40.5832)
  line L278 (63.7779, -40.5832) -> (63.6469, -40.597)
  line L279 (63.6469, -40.597) -> (63.516, -40.6126)
  line L280 (63.516, -40.6126) -> (63.4929, -40.6881)
  line L281 (63.4929, -40.6881) -> (63.4715, -40.7634)
  line L282 (63.4715, -40.7634) -> (63.4519, -40.8386)
  line L283 (63.4519, -40.8386) -> (63.4342, -40.9137)
  line L284 (63.4342, -40.9137) -> (63.4185, -40.9885)
  line L285 (63.4185, -40.9885) -> (63.4048, -41.0631)
  line L286 (63.4048, -41.0631) -> (63.3932, -41.1375)
  line L287 (63.3932, -41.1375) -> (63.384, -41.2116)
  line L288 (63.384, -41.2116) -> (63.3773, -41.2853)
  line L289 (63.3773, -41.2853) -> (63.3736, -41.3586)
  line L290 (63.3736, -41.3586) -> (63.3733, -41.4314)
  line L291 (63.3733, -41.4314) -> (63.3782, -41.5034)
  line L292 (63.3782, -41.5034) -> (63.4474, -41.9453)
  line L293 (63.4474, -41.9453) -> (63.2338, -41.9817)
  line L294 (63.2338, -41.9817) -> (63.0212, -42.0239)
  line L295 (63.0212, -42.0239) -> (62.8099, -42.0718)
  line L296 (62.8099, -42.0718) -> (62.5999, -42.1254)
  line L297 (62.5999, -42.1254) -> (62.4834, -41.6936)
  line L298 (62.4834, -41.6936) -> (62.4586, -41.6258)
  line L299 (62.4586, -41.6258) -> (62.4288, -41.5594)
  line L300 (62.4288, -41.5594) -> (62.3955, -41.494)
  line L301 (62.3955, -41.494) -> (62.3594, -41.4294)
  line L302 (62.3594, -41.4294) -> (62.3208, -41.3654)
  line L303 (62.3208, -41.3654) -> (62.28, -41.3022)
  line L304 (62.28, -41.3022) -> (62.2372, -41.2396)
  line L305 (62.2372, -41.2396) -> (62.1924, -41.1776)
  line L306 (62.1924, -41.1776) -> (62.1457, -41.1163)
  line L307 (62.1457, -41.1163) -> (62.0972, -41.0555)
  line L308 (62.0972, -41.0555) -> (62.047, -40.9954)
  line L309 (62.047, -40.9954) -> (61.9952, -40.9359)
  line L310 (61.9952, -40.9359) -> (61.8693, -40.9748)
  line L311 (61.8693, -40.9748) -> (61.7439, -41.0156)
  line L312 (61.7439, -41.0156) -> (61.6192, -41.0581)
  line L313 (61.6192, -41.0581) -> (61.6122, -41.1367)
  line L314 (61.6122, -41.1367) -> (61.607, -41.2148)
  line L315 (61.607, -41.2148) -> (61.6035, -41.2924)
  line L316 (61.6035, -41.2924) -> (61.6018, -41.3695)
  line L317 (61.6018, -41.3695) -> (61.6019, -41.446)
  line L318 (61.6019, -41.446) -> (61.604, -41.5218)
  line L319 (61.604, -41.5218) -> (61.6082, -41.597)
  line L320 (61.6082, -41.597) -> (61.6146, -41.6713)
  line L321 (61.6146, -41.6713) -> (61.6234, -41.7449)
  line L322 (61.6234, -41.7449) -> (61.635, -41.8174)
  line L323 (61.635, -41.8174) -> (61.6498, -41.8886)
  line L324 (61.6498, -41.8886) -> (61.6696, -41.958)
  line L325 (61.6696, -41.958) -> (61.8291, -42.3759)
  line L326 (61.8291, -42.3759) -> (61.6278, -42.4559)
  line L327 (61.6278, -42.4559) -> (61.4286, -42.5413)
  line L328 (61.4286, -42.5413) -> (61.2319, -42.6321)
  line L329 (61.2319, -42.6321) -> (61.0377, -42.7282)
  line L330 (61.0377, -42.7282) -> (60.8339, -42.3301)
  line L331 (60.8339, -42.3301) -> (60.7956, -42.269)
  line L332 (60.7956, -42.269) -> (60.7526, -42.2102)
  line L333 (60.7526, -42.2102) -> (60.7064, -42.1531)
  line L334 (60.7064, -42.1531) -> (60.6577, -42.0974)
  line L335 (60.6577, -42.0974) -> (60.6067, -42.0429)
  line L336 (60.6067, -42.0429) -> (60.5536, -41.9895)
  line L337 (60.5536, -41.9895) -> (60.4987, -41.9372)
  line L338 (60.4987, -41.9372) -> (60.4419, -41.8859)
  line L339 (60.4419, -41.8859) -> (60.3835, -41.8356)
  line L340 (60.3835, -41.8356) -> (60.3235, -41.7863)
  line L341 (60.3235, -41.7863) -> (60.2619, -41.7379)
  line L342 (60.2619, -41.7379) -> (60.1988, -41.6904)
  line L343 (60.1988, -41.6904) -> (60.0838, -41.7547)
  line L344 (60.0838, -41.7547) -> (59.9696, -41.8206)
  line L345 (59.9696, -41.8206) -> (59.8564, -41.8881)
  line L346 (59.8564, -41.8881) -> (59.866, -41.9665)
  line L347 (59.866, -41.9665) -> (59.8771, -42.044)
  line L348 (59.8771, -42.044) -> (59.8898, -42.1207)
  line L349 (59.8898, -42.1207) -> (59.9042, -42.1964)
  line L350 (59.9042, -42.1964) -> (59.9202, -42.2712)
  line L351 (59.9202, -42.2712) -> (59.9381, -42.3449)
  line L352 (59.9381, -42.3449) -> (59.9578, -42.4175)
  line L353 (59.9578, -42.4175) -> (59.9795, -42.489)
  line L354 (59.9795, -42.489) -> (60.0034, -42.559)
  line L355 (60.0034, -42.559) -> (60.0297, -42.6276)
  line L356 (60.0297, -42.6276) -> (60.0591, -42.6942)
  line L357 (60.0591, -42.6942) -> (60.0928, -42.758)
  line L358 (60.0928, -42.758) -> (60.3358, -43.1335)
  line L359 (60.3358, -43.1335) -> (60.1554, -43.2536)
  line L360 (60.1554, -43.2536) -> (59.9784, -43.3786)
  line L361 (59.9784, -43.3786) -> (59.8049, -43.5083)
  line L362 (59.8049, -43.5083) -> (59.6349, -43.6427)
  line L363 (59.6349, -43.6427) -> (59.3528, -43.2956)
  line L364 (59.3528, -43.2956) -> (59.3026, -43.2438)
  line L365 (59.3026, -43.2438) -> (59.2483, -43.1953)
  line L366 (59.2483, -43.1953) -> (59.1913, -43.1491)
  line L367 (59.1913, -43.1491) -> (59.132, -43.1047)
  line L368 (59.132, -43.1047) -> (59.0708, -43.062)
  line L369 (59.0708, -43.062) -> (59.0078, -43.0208)
  line L370 (59.0078, -43.0208) -> (58.9432, -42.981)
  line L371 (58.9432, -42.981) -> (58.877, -42.9427)
  line L372 (58.877, -42.9427) -> (58.8094, -42.9056)
  line L373 (58.8094, -42.9056) -> (58.7405, -42.8698)
  line L374 (58.7405, -42.8698) -> (58.6702, -42.8353)
  line L375 (58.6702, -42.8353) -> (58.5986, -42.802)
  line L376 (58.5986, -42.802) -> (58.4994, -42.8888)
  line L377 (58.4994, -42.8888) -> (58.4015, -42.977)
  line L378 (58.4015, -42.977) -> (58.3048, -43.0666)
  line L379 (58.3048, -43.0666) -> (58.3304, -43.1412)
  line L380 (58.3304, -43.1412) -> (58.3574, -43.2147)
  line L381 (58.3574, -43.2147) -> (58.3858, -43.2871)
  line L382 (58.3858, -43.2871) -> (58.4156, -43.3582)
  line L383 (58.4156, -43.3582) -> (58.4468, -43.428)
  line L384 (58.4468, -43.428) -> (58.4796, -43.4964)
  line L385 (58.4796, -43.4964) -> (58.514, -43.5633)
  line L386 (58.514, -43.5633) -> (58.55, -43.6287)